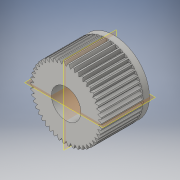
# Autodesk Inventor part: Servo Horn
Saved by Autodesk Inventor 2016 (Build 200138000, 138)
## iProperties
Created: 2016-02-11
Part Number: Servo Horn
Material: Generic
Document SubType Name: Modeling
Designer: RoksBot
Density: 1 g/cm^3
Appearance: Default
Author: RoksBot
Autodesk Inventor part; units mm, degrees
ref_plane "XY Plane" through (0, 0, 0) normal (0, 0, 1) x (1, 0, 0)
sketch "Sketch1" plane through (0, 0, 0) normal (0, 0, 1) x (1, 0, 0)
  circle A0 centre (0, 0) radius 2.8385
  circle A1 centre (0, 0) radius 1.1747
  dimension "d0" = 5.6769
  dimension "d1" = 2.3495
  constraints: 2 centre point, 2 coincident
  measures "d0" diameter of A0
  measures "d1" diameter of A1
extrude "Extrusion1" add sketch "Sketch1" along normal blind 3.81
sketch "Sketch2" plane through (0, 0, 3.81) normal (0, 0, 1) x (1, 0, 0)
  circle A0 centre (0, 0) radius 1.1747 projected
  circle A1 centre (0, 0) radius 2.8385 projected
  circle A2 centre (0, 0) radius 2.8385 projected
  line L0 (-0.1466, 2.8347) -> (0, 2.5807)
  line L1 (0, 2.5807) -> (0.1466, 2.8347)
  dimension "d4" = 0.254
  dimension "d5" = 60
  constraints: 4 end point, 4 point on circle, 1 equal length, 1 vertical alignment
  measures "d4" vertical distance of L1.end L0.end
  measures "d5" angle of L1 L0
extrude "Extrusion2" cut sketch "Sketch2" against normal blind 3.302 contours L1 L0 A1 picked at (0.0652, 2.7512)
pattern_circular "Circular Pattern1" count 46 over 360 about axis through (0, 0, 0) along (0, 0, 1) of "Extrusion2"
ref_plane "Work Plane1" through (0, 0, 0) normal (1, 0, 0) x (0, 1, 0)
ref_plane "Work Plane2" through (0, 0, 0) normal (0, 1, 0) x (-1, 0, 0)
body "Solid1"
